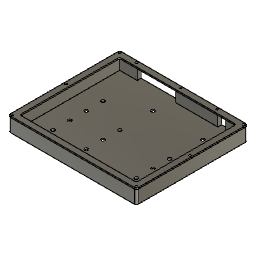
BFO9000-Case v4 (Autodesk Fusion 360 design; units mm, degrees)
Autodesk Fusion 360 part; units mm, degrees
sketch "Layout" plane through (0, 0, 0) normal (0, 0, 1) x (1, 0, 0) in component "Case"
  line L0 (0, 0) -> (133, 0)
  line L1 (133, 0) -> (133, 114)
  line L2 (133, 114) -> (0, 114)
  line L3 (0, 114) -> (0, 0)
  circle A0 centre (19, 95) radius 2
  circle A1 centre (38, 95) radius 2
  circle A2 centre (57, 95) radius 2
  circle A3 centre (76, 95) radius 2
  circle A4 centre (95, 95) radius 2
  circle A5 centre (114, 95) radius 2
  circle A6 centre (19, 76) radius 2
  circle A7 centre (38, 76) radius 2
  circle A8 centre (57, 76) radius 2
  circle A9 centre (76, 76) radius 2
  circle A10 centre (95, 76) radius 2
  circle A11 centre (114, 76) radius 2
  circle A12 centre (19, 57) radius 2
  circle A13 centre (38, 57) radius 2
  circle A14 centre (57, 57) radius 2
  circle A15 centre (76, 57) radius 2
  circle A16 centre (95, 57) radius 2
  circle A17 centre (114, 57) radius 2
  circle A18 centre (19, 38) radius 2
  circle A19 centre (38, 38) radius 2
  circle A20 centre (57, 38) radius 2
  circle A21 centre (76, 38) radius 2
  circle A22 centre (95, 38) radius 2
  circle A23 centre (114, 38) radius 2
  circle A24 centre (19, 19) radius 2
  circle A25 centre (38, 19) radius 2
  circle A26 centre (57, 19) radius 2
  circle A27 centre (76, 19) radius 2
  circle A28 centre (95, 19) radius 2
  circle A29 centre (114, 19) radius 2
  line L4 (-2, -2) -> (135, -2)
  line L5 (135, -2) -> (135, 116)
  line L6 (135, 116) -> (-2, 116)
  line L7 (-2, 116) -> (-2, -2)
  line L8 (-4.4, -6.4) -> (137.4, -6.4)
  line L9 (139.4, -4.4) -> (139.4, 118.4)
  line L10 (137.4, 120.4) -> (-4.4, 120.4)
  line L11 (-6.4, 118.4) -> (-6.4, -4.4)
  line L12 (135, 116) -> (139.4, 120.4) construction
  line L13 (-2, 116) -> (-6.4, 120.4) construction
  line L14 (-6.4, -6.4) -> (-2, -2) construction
  line L15 (135, -2) -> (139.4, -6.4) construction
  circle A30 centre (-4.2, 118.2) radius 1.23
  circle A31 centre (137.2, 118.2) radius 1.23
  circle A32 centre (137.2, -4.2) radius 1.23
  circle A33 centre (-4.2, -4.2) radius 1.23
  line L16 (133, 114) -> (0, 0) construction
  line L17 (0, 114) -> (133, 0) construction
  line L18 (66.5, 57) -> (133, 57) construction
  line L19 (66.5, 57) -> (0, 57) construction
  line L20 (66.5, 57) -> (66.5, 114) construction
  line L21 (66.5, 57) -> (66.5, 0) construction
  line L22 (137.2, 118.2) -> (137.2, -4.2) construction
  line L23 (-4.2, 118.2) -> (-4.2, -4.2) construction
  line L24 (135, 57) -> (139.4, 57) construction
  line L25 (-2, 57) -> (-6.4, 57) construction
  circle A34 centre (137.2, 57) radius 1.23
  circle A35 centre (-4.2, 57) radius 1.23
  arc A36 (137.4, -6.4) -> (139.4, -4.4) centre (137.4, -4.4) ccw
  arc A37 (139.4, 118.4) -> (137.4, 120.4) centre (137.4, 118.4) ccw
  arc A38 (-4.4, 120.4) -> (-6.4, 118.4) centre (-4.4, 118.4) ccw
  arc A39 (-6.4, -4.4) -> (-4.4, -6.4) centre (-4.4, -4.4) ccw
  line L26 (135, 116) -> (135, 120.4) construction
  line L27 (119, 116) -> (119, 120.4)
  line L28 (110, 116) -> (110, 120.4)
  line L29 (62, 116) -> (62, 120.4)
  line L30 (18, 116) -> (18, 120.4)
  line L31 (0, 114) -> (0, 120.4)
  circle A40 centre (122, 118.2) radius 1.23
  circle A41 centre (107, 118.2) radius 1.23
  circle A42 centre (65, 118.2) radius 1.23
  circle A43 centre (15, 118.2) radius 1.23
  dimension "d3" = 133
  dimension "d4" = 114
  dimension "BigHoleDiameter" = 4
  dimension "d6" = 19
  dimension "d7" = 19
  dimension "d10" = 19
  dimension "d11" = -19
  dimension "BreathingSpace" = 2
  dimension "d13" = 133
  dimension "d17" = 2.46
  dimension "d18" = 2.46
  dimension "d19" = 2.46
  dimension "d20" = 2.46
  dimension "d21" = 2.46
  dimension "CornerRadius" = 2
  dimension "d25" = 2
  dimension "d26" = 2
  dimension "d27" = 2
  dimension "d28" = 4.4
  dimension "d29" = 16
  dimension "d30" = 9
  dimension "d31" = 48
  dimension "d32" = 44
  dimension "d33" = 19
  dimension "d55" = 2.46
  dimension "d56" = 3
  dimension "d57" = 2.46
  dimension "d58" = 2.46
  dimension "d59" = 2.46
  dimension "d60" = 3
  dimension "d61" = 3
  dimension "d62" = 3
  constraint horizontal L0
  constraint vertical L1
  constraint horizontal L2
  constraint vertical L3
  constraint coincident L0.start L3.end
  constraint midpoint L13 A30.centre
  constraint midpoint L12 A31.centre
  constraint midpoint L15 A32.centre
  constraint midpoint L14 A33.centre
  constraint midpoint L17 L18.start
  constraint midpoint L1 L18.end
  constraint midpoint L3 L19.end
  constraint midpoint L2 L20.end
  constraint midpoint L0 L21.end
  constraint coincident A31.centre L22.start
  constraint coincident A32.centre L22.end
  constraint coincident A30.centre L23.start
  constraint coincident A33.centre L23.end
  constraint midpoint L5 L24.start
  constraint midpoint L7 L25.start
  constraint symmetric L20 A34 A35
  constraint parallel L0 L8
  constraint parallel L1 L9
  constraint parallel L2 L10
  constraint parallel L3 L11
  constraint coincident L9 L24.end
  constraint coincident L15.end L9
  constraint coincident L15.end L8
  constraint tangent L9 A36
  constraint tangent L8 A36
  constraint coincident L12.end L9
  constraint coincident L12.end L10
  constraint tangent L9 A37
  constraint tangent L10 A37
  constraint coincident L11 L25.end
  constraint coincident L13.end L11
  constraint coincident L13.end L10
  constraint tangent L11 A38
  constraint tangent L10 A38
  constraint coincident L14.start L8
  constraint coincident L14.start L11
  constraint tangent L8 A39
  constraint tangent L11 A39
  constraint coincident L23 A35.centre
  constraint coincident L10 L26.end
  constraint perpendicular L10 L26
  constraint coincident L6 L27.start
  constraint coincident L10 L27.end
  constraint perpendicular L10 L27
  constraint coincident L6 L28.start
  constraint coincident L10 L28.end
  constraint perpendicular L10 L28
  constraint coincident L6 L29.start
  constraint coincident L10 L29.end
  constraint perpendicular L10 L29
  constraint coincident L6 L30.start
  constraint coincident L10 L30.end
  constraint perpendicular L10 L30
  constraint coincident L10 L31.end
  constraint perpendicular L10 L31
  constraint midpoint L22 A34.centre
  measures "d3" distance of L0.start L0.end
  measures "d4" distance of L0.start L2.end
  measures "BigHoleDiameter" diameter of A0
  measures "d6" distance of L3 A0.centre
  measures "d7" distance of L2 A0.centre
  measures "d13" distance of L1 L3
  measures "d17" diameter of A30
  measures "d18" diameter of A31
  measures "d19" diameter of A32
  measures "d20" diameter of A33
  measures "d21" diameter of A34
  measures "CornerRadius" radius of A36
  measures "d25" radius of A37
  measures "d26" radius of A38
  measures "d27" radius of A39
  measures "d28" distance of L6 L10
  measures "d29" distance of L26 L27
  measures "d30" distance of L27 L28
  measures "d31" distance of L28 L29
  measures "d32" distance of L29 L30
  measures "d55" diameter of A40
  measures "d56" distance of L27 A40.centre
  measures "d57" diameter of A41
  measures "d58" diameter of A42
  measures "d59" diameter of A43
  measures "d60" distance of L30 A43.centre
  measures "d61" distance of L29 A42.centre
  measures "d62" distance of L28 A41.centre
extrude "Extrude1" add sketch "Layout" along normal blind 1.5 contours L0 L1 L2 L3 | A0 | A1 | A3 | A4 | A7 | A8 | A9 | A10 | A11 | A13 | A15 | A16 | A19 | A21 | A22 | A25 | A27 | A28 | L4 L5 L6 L7 | L6 L10 L27 L28 | L6 L10 L29 L30 makes body 1 in component "Case"
extrude "Extrude2" add sketch "Layout" along normal blind 15 contours L4 L5 L6 L7 L8 L9 L10 L11 A36 A37 A38 A39 L27 L31 | L6 L10 L30 L31 | L6 L10 L28 L29 | A30 | A31 | A32 | A33 | A34 | A35 | A40 | A41 | A42 | A43 bodies 1 in component "Case"
extrude "Extrude3" cut sketch "Layout" against normal blind 11.5 from surface at 15 contours A30 | A31 | A32 | A33 | A34 | A35 | A40 | A41 | A42 | A43 bodies 1 in component "Case"
extrude "Extrude4" add sketch "Layout" along normal blind 1.5 from surface at 15 separate body contours L4 L5 L6 L7 | L4 L5 L6 L7 L8 L9 L10 L11 A36 A37 A38 A39 L27 L31 | L6 L10 L30 L31 | L6 L10 L27 L28 | L6 L10 L29 L30 | L6 L10 L28 L29 | A40 makes body 2 in component "Case"
ref_plane "WorkPlane1" through (0, 57, 0) normal (0, 1, 0) x (0, 0, 1) in component "Case"
fillet "Fillet2" radius 2 1 edges at (133, 0, 15.75) on bodies 2 in component "Case"
fillet "Fillet2" radius 2 1 edges at (0, 0, 15.75) on bodies 2 in component "Case"
fillet "Fillet2" radius 2 1 edges at (0, 114, 15.75) on bodies 2 in component "Case"
fillet "Fillet2" radius 2 1 edges at (133, 114, 15.75) on bodies 2 in component "Case"
component "Case" placed x (1, 0, 0) y (0, 1, 0) z (0, 0, 1) at (0, 0, 0)
equation "NumColumns = 7"
equation "NumRows = 6"
equation "d3 = ( NumColumns * 19 ) * 1 mm"
equation "d4 = ( NumRows * 19 ) * 1 mm"
equation "d8 = NumColumns - 1"
equation "d9 = NumRows - 1"
equation "EdgeWidth = 4.4 mm"
equation "ScrewSize = 2.46 mm"
equation "d25 = CornerRadius"
equation "d26 = CornerRadius"
equation "d27 = CornerRadius"
equation "d28 = EdgeWidth"
equation "d29 = 14 mm + BreathingSpace"
equation "BaseHeight = 1.5 mm"
equation "Height = 13.5 mm"
equation "d36 = BaseHeight"
equation "d38 = BaseHeight + Height"
equation "d41 = -Height + 2 mm"
equation "d55 = ScrewSize"
equation "d57 = ScrewSize"
equation "d58 = ScrewSize"
equation "d59 = ScrewSize"
named bodies: "Base", "UpperPlate"
